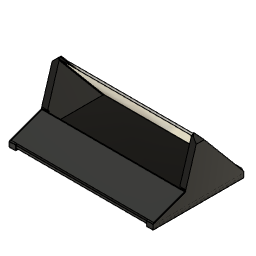
tablet-hud (Autodesk Fusion 360 design; units mm, degrees)
Autodesk Fusion 360 part; units mm, degrees
note: some values were not read from the file. Chosen so that the rebuilt part matches the saved one: a direction. Set by a fixed rule: which sketch regions a step uses.
sketch "Sketch1" plane through (0, 0, 0) normal (0, 0, 1) x (1, 0, 0)
  line L0 (10, 0) -> (235, 0)
  line L1 (245, 10) -> (245, 150)
  line L2 (235, 160) -> (10, 160)
  line L3 (0, 150) -> (0, 10)
  arc A0 (10, 160) -> (0, 150) centre (10, 150) ccw
  arc A1 (0, 10) -> (10, 0) centre (10, 10) ccw
  arc A2 (235, 0) -> (245, 10) centre (235, 10) ccw
  arc A3 (245, 150) -> (235, 160) centre (235, 150) ccw
  point P0 (245, 0)
  point P1 (0, 160)
  dimension "d14" = 245
  dimension "d15" = 160
  dimension "d16" = 10
  constraint horizontal L0
  constraint vertical L1
  constraint horizontal L2
  constraint vertical L3
  constraint coincident P1 L2
  constraint coincident P1 L3
  constraint tangent L2 A0
  constraint tangent L3 A0
  constraint coincident origin L0
  constraint coincident origin L3
  constraint tangent L0 A1
  constraint tangent L3 A1
  constraint equal A0 A1
  constraint coincident P0 L0
  constraint coincident P0 L1
  constraint tangent L0 A2
  constraint tangent L1 A2
  constraint equal A0 A2
  constraint tangent L1 A3
  constraint tangent L2 A3
  constraint equal A0 A3
  measures "d14" distance of origin P0
  measures "d15" distance of origin P1
  measures "d16" radius of A0
extrude "Extrude1" add sketch "Sketch1" along normal blind 5.85 makes body 1
fillet "Fillet1" radius 2 8 edges at (245, 80, 0) (242.0711, 157.0711, 0) (122.5, 160, 0) (2.9289, 157.0711, 0) (0, 80, 0) (2.9289, 2.9289, 0) (122.5, 0, 0) (242.0711, 2.9289, 0) on bodies 1
sketch "Sketch9" plane through (0, 0, 5.85) normal (0, 0, 1) x (-1, 0, 0)
  arc A0 (-245, -150) -> (-235, -160) centre (-235, -150) ccw
  line L0 (-235, -160) -> (-10, -160)
  arc A1 (-10, -160) -> (0, -150) centre (-10, -150) ccw
  line L1 (0, -150) -> (0, -10)
  arc A2 (0, -10) -> (-10, 0) centre (-10, -10) ccw
  line L2 (-10, 0) -> (-235, 0)
  arc A3 (-235, 0) -> (-245, -10) centre (-235, -10) ccw
  line L3 (-245, -10) -> (-245, -150)
  line L4 (-236, -9) -> (-9, -9)
  line L5 (-9, -9) -> (-9, -151)
  line L6 (-9, -151) -> (-236, -151)
  line L7 (-236, -151) -> (-236, -9)
  dimension "d89" = 9
  dimension "d90" = 9
  dimension "d91" = 9
  dimension "d92" = 9
  constraint horizontal L4
  constraint vertical L5
  constraint horizontal L6
  constraint vertical L7
  measures "d89" distance of L0 L6
  measures "d90" distance of L2 L4
  measures "d91" distance of L1 L5
  measures "d92" distance of L3 L7
ref_plane "WorkPlane1" through (122.5, 151, 5.85) normal (0, 0.766044, 0.642788) x (1, 0, 0)
sketch "Sketch2" plane through (122.5, 154.7186, 1.4184) normal (0, 0.766044, 0.642788) x (-1, 0, 0)
  line L0 (-112.5, 0) -> (112.5, 0) construction
  line L1 (-114, 5.7851) -> (114, 5.7851)
  line L2 (114, 5.7851) -> (114, 199.7851)
  line L3 (114, 199.7851) -> (-114, 199.7851)
  line L4 (-114, 199.7851) -> (-114, 5.7851)
  line L5 (113.5, 5.7851) -> (-113.5, 5.7851)
  line L6 (0, 199.7851) -> (0, 5.7851) construction
  dimension "d22" = 228
  dimension "d23" = 194
  constraint vertical L2
  constraint horizontal L3
  constraint vertical L4
  constraint collinear L1 L5
  constraint midpoint L3 L6.start
  constraint midpoint L1 L6.end
  constraint coincident origin L6
  measures "d22" distance of L1.start L1.end
  measures "d23" distance of L1.start L3.end
extrude "Extrude2" add sketch "Sketch2" along normal blind 3.2 separate body makes body 2
ref_plane "WorkPlane2" through (122.5, 0, 5.85) normal (0, -0.34202, 0.939693) x (1, 0, 0)
sketch "Sketch3" plane through (122.5, 0, 5.85) normal (0, -0.34202, 0.939693) x (1, 0, 0)
  line L0 (-112.5, 0) -> (112.5, 0) construction
  line L1 (-122.5, 0) -> (122.5, 0)
  line L2 (122.5, 0) -> (122.5, 60)
  line L3 (122.5, 60) -> (-122.5, 60)
  line L4 (-122.5, 60) -> (-122.5, 0)
  dimension "d27" = 245
  dimension "d28" = 60
  constraint horizontal L1
  constraint vertical L2
  constraint horizontal L3
  constraint vertical L4
  constraint midpoint L0 L1
  measures "d27" distance of L1.start L1.end
  measures "d28" distance of L1.start L3.end
extrude "Extrude3" add sketch "Sketch3" along normal blind 2 separate body makes body 3
chamfer "Chamfer1" distance 1.8 angle 45 2 edges at (122.5, -0.684, 7.7294) (122.5, 55.6975, 28.2506) on bodies 3
ref_plane "WorkPlane3" through (122.5, 80, 2.925) normal (-1, 0, 0) x (0, -1, 0)
sketch "Sketch7" plane through (122.5, 80, 2.925) normal (-1, 0, 0) x (0, 1, 0)
  line L0 (-80, 0.925) -> (-80, -2.925) construction
  arc A0 (-78, 2.925) -> (-80, 0.925) centre (-78, 0.925) ccw construction
  line L1 (-80, -2.925) -> (-855.2761, -200.275) construction
  line L2 (70, -2.925) -> (-70, -2.925) construction
  line L3 (70, -2.925) -> (80, -2.925) construction
  line L4 (80, 0.925) -> (80, -2.925) construction
  line L5 (71, -2.925) -> (-53.7008, -151.5376) construction
  line L6 (-8, -2.925) -> (-3.7197, -91.9725)
  line L7 (-3.7197, -91.9725) -> (-855.2761, -200.275)
  line L8 (-3.7197, -91.9725) -> (-92.1577, -103.2202) construction
  line L9 (-92.1577, -103.2202) -> (-45.7986, -142.1201) construction
  line L10 (-8, -2.925) -> (38.3591, -41.8249) construction
  line L11 (-53.7008, -151.5376) -> (-45.7986, -142.1201) construction
  line L12 (71, -2.925) -> (-855.2761, -200.275)
  dimension "d79" = 800
  dimension "d80" = 203.2
  dimension "d81" = 88
  constraint coincident L0.end L1.start
  constraint coincident L2 L6.start
  constraint coincident L5 L6.end
  constraint parallel L7 L8
  constraint equal L6 L8
  constraint coincident L5 L10.end
  constraint perpendicular L5 L10
  constraint equal L9 L10
  constraint coincident L5.end L11.start
  constraint collinear L5 L11
  constraint perpendicular L9 L11
  constraint coincident L5.start L12.start
  measures "d79" distance of L0.end L1.end
  measures "d80" vertical distance of A0.start L1.end
  measures "d81" distance of L3.end L6.start
sketch "Sketch8" plane through (0, 91.491, 76.7701) normal (0, -0.766044, -0.642788) x (1, 0, 0)
  line L0 (236.5, -92.5796) -> (236.5, 101.4204)
  line L1 (236.5, 101.4204) -> (8.5, 101.4204)
  line L2 (8.5, 101.4204) -> (8.5, -92.5796)
  line L3 (8.5, -92.5796) -> (236.5, -92.5796)
  line L4 (122.5, 23.6637) -> (8.5, 23.6637) construction
  line L5 (122.5, 23.6637) -> (236.5, 23.6637) construction
  line L6 (236.5, 25.6637) -> (8.5, 25.6637)
  point P0 (122.5, 23.6637)
  dimension "d86" = 2
  constraint coincident P0 L4.start
  constraint coincident L2 L4.end
  constraint perpendicular L2 L4
  constraint coincident L0 L5.end
  constraint perpendicular L0 L5
  constraint coincident L0 L6.start
  constraint coincident L2 L6.end
  constraint perpendicular L2 L6
  measures "d86" distance of L4 L6
extrude "Extrude11" cut sketch "Sketch8" against normal blind 3.2 contours L0 L1 L2 L6 bodies 2
sketch "Sketch4" plane through (0, 0, 0) normal (-1, 0, 0) x (0, -1, 0)
  line L0 (-150, 2) -> (-10, 2)
  line L1 (-10, 2) -> (-10, 5.85)
  line L2 (-10, 5.85) -> (-150, 5.85)
  line L3 (-150, 5.85) -> (-150, 2)
  line L4 (-151, 5.85) -> (-74.9947, 96.4296) construction
  line L5 (-77.446, 98.4865) -> (-153.4513, 7.9069) construction
  line L6 (-153.4513, 7.9069) -> (-151, 5.85) construction
  line L7 (-160, 2) -> (-160, 5.85) construction
  line L8 (-150, 0) -> (-10, 0) construction
  line L9 (0, 2) -> (0, 5.85) construction
  line L10 (-54.0061, 27.635) -> (-56.3132, 26.5591) construction
  line L11 (-56.3132, 26.5591) -> (-56.3816, 26.3712) construction
  line L12 (-56.3816, 26.3712) -> (0, 5.85) construction
  line L13 (0, 5.85) -> (0.0684, 6.0379) construction
  line L14 (0.0684, 6.0379) -> (-1.0074, 8.345) construction
  line L15 (-1.0074, 8.345) -> (-54.0061, 27.635) construction
  line L16 (-138.7943, 27.2414) -> (-154.6513, 8.3437)
  line L17 (-154.6513, 8.3437) -> (-154.6513, -1.2)
  line L18 (-154.6513, -1.2) -> (1.2, -1.2)
  line L19 (1.2, -1.2) -> (1.2, 7.5416)
  line L20 (1.2, 7.5416) -> (-1.0074, 8.345)
  line L21 (-1.0074, 8.345) -> (-54.0061, 27.635)
  line L22 (-138.7943, 27.2414) -> (-79.0206, 98.4769)
  line L23 (-74.9947, 96.4296) -> (-77.446, 98.4865)
  line L24 (-77.446, 98.4865) -> (-79.0206, 98.4769)
  line L25 (-74.9947, 96.4296) -> (-54.0061, 27.635)
  line L26 (-74.9947, 96.4296) -> (-77.446, 98.4865)
  dimension "d32" = 1.2
  dimension "d33" = 1.2
  dimension "d34" = 1.2
  dimension "d35" = 1.2
  constraint parallel L5 L16
  constraint perpendicular L17 L18
  constraint perpendicular L18 L19
  constraint coincident L14.end L15.start
  constraint parallel L15 L20
  constraint coincident L10.start L15.end
  constraint parallel L16 L22
  constraint coincident L4.end L23.start
  constraint coincident L5.start L23.end
  measures "d32" distance of L9 L19
  measures "d33" distance of L8 L18
  measures "d34" distance of L5.end L17
  measures "d35" distance of L5 L16
extrude "Extrude4" add sketch "Sketch4" along normal blind 1.2 separate body contours L0 L1 L2 L3 | L16 L17 L18 L19 L20 L21 L22 L23 L24 L25 L26 makes body 4
sketch "Sketch5" plane through (0, 0, 0) normal (-1, 0, 0) x (0, -1, 0)
  line L0 (0.0684, 6.0379) -> (-1.0074, 8.345)
  line L1 (0, 5.85) -> (0.0684, 6.0379)
  line L2 (-56.3816, 26.3712) -> (0, 5.85)
  line L3 (0, 2) -> (0, 5.85)
  line L4 (-150, 0) -> (-10, 0)
  line L5 (-56.3132, 26.5591) -> (-56.3816, 26.3712)
  line L6 (-54.0061, 27.635) -> (-56.3132, 26.5591)
  line L7 (-160, 2) -> (-160, 5.85)
  line L8 (-77.446, 98.4865) -> (-153.4513, 7.9069)
  line L9 (-153.4513, 7.9069) -> (-151, 5.85)
  line L10 (-151, 5.85) -> (-74.9947, 96.4296)
  line L11 (-160, 2) -> (-160, 0)
  line L12 (-160, 0) -> (-150, 0)
  line L13 (-10, 0) -> (0, 0)
  line L14 (0, 0) -> (0, 2)
  line L15 (-54.0061, 27.635) -> (1.2, 7.5416)
  line L16 (1.2, 7.5416) -> (1.2, -1.2)
  line L17 (1.2, -1.2) -> (-154.6513, -1.2)
  line L18 (-154.6513, -1.2) -> (-154.6513, 8.3437)
  line L19 (-154.6513, 8.3437) -> (-79.0206, 98.4769)
  line L20 (-160, 5.85) -> (0, 5.85) construction
  line L21 (-3.297, 7.05) -> (-149.9931, 7.05) construction
  line L22 (-3.297, 7.05) -> (-3.297, 5.85)
  line L23 (-13.297, 5.85) -> (-13.297, 10.6897)
  line L24 (-13.297, 5.85) -> (-3.297, 5.85)
  line L25 (-59.0472, 26.0644) -> (-47.3951, 21.8234)
  line L26 (-47.3951, 21.8234) -> (-46.9846, 22.951)
  line L27 (-149.9931, 7.05) -> (-149.9931, 5.85)
  line L28 (-74.577, 95.0605) -> (-148.4266, 7.05)
  line L29 (-148.4266, 7.05) -> (-138.4266, 7.05)
  line L30 (-138.4266, 7.05) -> (-138.4266, 5.85)
  line L31 (-138.4266, 5.85) -> (-149.9931, 5.85)
  line L32 (-59.0472, 26.0644) -> (-58.3256, 28.0473)
  line L33 (-56.3816, 26.3712) -> (-56.792, 25.2436) construction
  line L34 (-148.4266, 7.05) -> (-149.4335, 5.85)
  line L35 (-52.8616, 31.4982) -> (-56.6024, 29.7538)
  line L36 (-56.6024, 29.7538) -> (-57.6637, 26.8379)
  line L37 (-56.3816, 26.3712) -> (-57.6637, 26.8379)
  line L38 (-75.4971, 93.964) -> (-56.7267, 32.4401)
  line L39 (-58.3256, 28.0473) -> (-56.7267, 32.4401)
  line L40 (-79.0206, 98.4769) -> (-77.446, 98.4865)
  line L41 (-77.446, 98.4865) -> (-74.9947, 96.4296)
  line L42 (-74.9947, 96.4296) -> (-54.0061, 27.635)
  line L43 (-153.4513, 7.9069) -> (-153.4513, 5.85)
  line L44 (-154.6513, 5.85) -> (-153.4513, 5.85)
  line L45 (-153.4513, 5.85) -> (-149.9931, 5.85)
  line L46 (-13.297, 5.85) -> (-149.4335, 5.85)
  line L47 (-74.1276, 89.4752) -> (-79.2636, 89.4752)
  dimension "d39" = 1.2
  dimension "d40" = 10
  dimension "d43" = 1.2
  dimension "d44" = 10
  dimension "d45" = 1.2
  dimension "d46" = 10
  dimension "d47" = 2.4
  dimension "d99" = 1.2
  dimension "d100" = 9
  constraint coincident L7.start L11.start
  constraint vertical L11
  constraint coincident L4.start L12.end
  constraint perpendicular L11 L12
  constraint coincident L4.end L13.start
  constraint coincident L13.end L14.start
  constraint coincident L3.start L14.end
  constraint coincident L7.end L20.start
  constraint coincident L1.start L2.end
  constraint coincident L2 L21.start
  constraint coincident L10 L21.end
  constraint perpendicular L16 L21
  constraint coincident L20 L22.end
  constraint perpendicular L20 L22
  constraint coincident L20 L23.start
  constraint coincident L2 L23.end
  constraint perpendicular L21 L23
  constraint parallel L2 L25
  constraint coincident L2 L26.end
  constraint perpendicular L2 L26
  constraint coincident L20 L27.end
  constraint perpendicular L20 L27
  constraint coincident L21 L28.end
  constraint perpendicular L9 L28
  constraint parallel L21 L29
  constraint coincident L20 L30.end
  constraint perpendicular L20 L30
  constraint perpendicular L25 L32
  constraint coincident L2.start L5.end
  constraint coincident L25 L33.end
  constraint perpendicular L25 L33
  constraint parallel L28 L34
  constraint coincident L31 L34.end
  constraint perpendicular L33 L37
  constraint coincident L28 L38.start
  constraint collinear L32 L39
  constraint coincident L42 L28.start
  constraint coincident L8.end L9.start
  constraint coincident L20 L43.end
  constraint perpendicular L20 L43
  constraint coincident L18 L44.start
  constraint coincident L20 L44.start
  constraint parallel L38 L42
  constraint coincident L38 L47.start
  constraint coincident L28 L47.end
  constraint horizontal L47
  measures "d39" distance of L20 L21
  measures "d40" distance of L22.end L23.start
  measures "d43" distance of L2 L25
  measures "d44" distance of L2.start L26
  measures "d45" distance of L10 L28
  measures "d46" distance of L28.end L29.end
  measures "d47" distance of L5 L32
  measures "d99" distance of L38 L42
  measures "d100" distance of L40 L47.end
extrude "Extrude5" add sketch "Sketch5" against normal up to surface (10 mm away) contours L0 L1 L3 L4 L12 L13 L14 L15 L16 L17 L18 bodies 4
extrude "Extrude6" add sketch "Sketch5" against normal up to surface (8.5 mm away) contours L8 L9 L10 L41 | L10 L27 L45 | L9 L43 L45 bodies 4
extrude "Extrude7" add sketch "Sketch5" against normal blind 10 contours L10 L27 L28 L31 L34 L42 | L8 L18 L19 L40 L43 L44 bodies 4
extrude "Extrude9" add sketch "Sketch5" against normal blind 9 contours L2 L22 L23 L24 | L2 L25 L26 L28 L32 L35 L36 L37 L38 L39 L42 | L2 L23 L25 L26 L28 L29 L30 L32 L38 L39 L46 L47 | L28 L38 L47 | L29 L30 L31 L34 L46 bodies 4
chamfer "Chamfer2" distance 9 angle 45 1 edges at (-1.2, 78.2333, 98.4817) on bodies 4
fillet "Fillet2" radius 0.8 2 edges at (9.25, 77.446, 98.4865) (9.25, 74.9947, 96.4296) on bodies 4
mirror "Mirror1" about plane through (122.5, 80, 2.925) normal (-1, 0, 0) of bodies 4 makes body 5
sketch "Sketch6" plane through (-1.2, 0, 0) normal (-1, 0, 0) x (0, -1, 0)
  line L0 (1.2, 7.5416) -> (-54.0061, 27.635)
  line L1 (-86.6116, 89.4303) -> (-154.6513, 8.3437)
  line L2 (-154.6513, 8.3437) -> (-154.6513, -1.2)
  line L3 (-154.6513, -1.2) -> (1.2, -1.2)
  line L4 (1.2, -1.2) -> (1.2, 7.5416)
  line L5 (-150, 5.85) -> (-10, 5.85) construction
  line L6 (-150, 0) -> (-10, 0) construction
  line L7 (-80, 4.85) -> (-80, 0) construction
  line L8 (-83, 0) -> (-77, 0)
  arc A0 (-77, 0) -> (-77, 4.85) centre (-77, 2.425) ccw
  line L9 (-77, 4.85) -> (-83, 4.85)
  arc A1 (-83, 4.85) -> (-83, 0) centre (-83, 2.425) ccw
  line L10 (-83, 2.425) -> (-77, 2.425) construction
  line L11 (-54.0061, 27.635) -> (-72.8849, 89.5142)
  line L12 (-72.8849, 89.5142) -> (-86.6116, 89.4303)
  point P0 (-80, 2.425)
  dimension "d62" = 1
  dimension "d63" = 6
  constraint midpoint L6 L7.end
  constraint tangent L8 A0
  constraint tangent A0 L9
  constraint parallel L8 L9
  constraint tangent L9 A1
  constraint tangent L8 A1
  constraint perpendicular L7 L10
  constraint midpoint L7 P0
  constraint midpoint L10 P0
  constraint vertical L7
  constraint collinear L6 L8
  measures "d62" distance of L5 L7.start
  measures "d63" distance of A1.centre A0.centre
extrude "Extrude10" cut sketch "Sketch6" against normal blind 1.2 contours L8 A0 L9 A1 bodies 4
equation "tablet_thickness = 5.85 mm"
equation "tablet_width = 245 mm"
equation "tablet_height = 160 mm"
equation "tablet_corner_radius = 10 mm" comment "oversize to play it safe"
equation "mirror_thickness = 3.2 mm"
equation "mirror_width = 228 mm" comment "should be less than tablet width (aim for screen width)"
equation "mirror_height = 194 mm" comment "this doesn't do anything"
equation "mirror_angle = 50 deg" comment "angle between tablet and mirror, adjust for preference"
equation "shield_height = 60 mm"
equation "shield_angle = 20 deg"
equation "d14 = tablet_width"
equation "d15 = tablet_height"
equation "d16 = tablet_corner_radius"
equation "d17 = tablet_thickness"
equation "d21 = -mirror_angle"
equation "d22 = mirror_width"
equation "d23 = mirror_height"
equation "d24 = mirror_thickness"
equation "d26 = shield_angle"
equation "d27 = tablet_width"
equation "d28 = shield_height"
equation "d68 = display_side_bezel"
equation "display_bottom_bezel = 9 mm"
equation "display_side_bezel = 9 mm"
equation "display_height_scale = 0.55"
equation "eyes_distance = 800 mm" comment "line of sight from closest edge of tablet to eyes"
equation "eyes_elevation = 8\"" comment "elevation from tablet plane to eyes"
equation "d79 = eyes_distance"
equation "d80 = eyes_elevation"
equation "d81 = tablet_height * display_height_scale"
equation "d89 = display_bottom_bezel"
equation "d90 = display_bottom_bezel"
equation "d91 = display_side_bezel"
equation "d92 = display_side_bezel"
equation "d98 = -display_side_bezel"
equation "d100 = display_side_bezel"
named bodies: "Tablet", "Mirror", "Shield", "Left Wall", "Right Wall"
